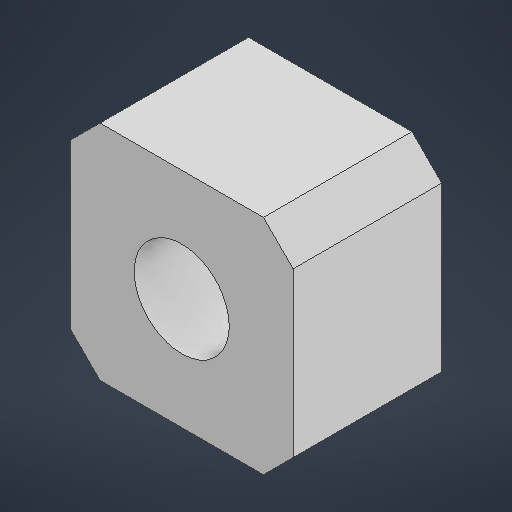
# Autodesk Inventor part: EndEffector_holder_Touch
Saved by Autodesk Inventor 2025.2 (Build 292293000, 293)
## iProperties
Created: 2025-07-03
Part Number: EndEffector_holder_Touch
Material: Generic
Document SubType Name: Modeling
Designer: Tiago
Density: 1 g/cm^3
Appearance: Default
Author: Tiago
Autodesk Inventor part; units mm, degrees
ref_plane "YZ Plane" through (0, 0, 0) normal (1, 0, 0) x (0, 1, 0)
ref_plane "XZ Plane" through (0, 0, 0) normal (0, 1, 0) x (-1, 0, 0)
ref_plane "XY Plane" through (0, 0, 0) normal (0, 0, 1) x (1, 0, 0)
sketch "Sketch1" plane through (0, 0, 0) normal (0, 0, 1) x (1, 0, 0)
  circle A0 centre (0, 0) radius 1.6
  line L0 (-3.75, -3.75) -> (3.75, -3.75)
  line L1 (3.75, -3.75) -> (3.75, 3.75)
  line L2 (3.75, 3.75) -> (-3.75, 3.75)
  line L3 (-3.75, 3.75) -> (-3.75, -3.75)
  point P0 (3.75, 0)
  point P1 (0, 3.75)
  dimension "d0" = 3.2
  dimension "d1" = 7.5
  dimension "d2" = 7.5
  constraints: 8 end point, 2 midpoint, 2 parallel, 1 centre point, 1 coincident, 1 horizontal, 1 horizontal alignment, 1 perpendicular, 1 vertical alignment
  measures "d0" diameter of A0
  measures "d1" distance of L0.end L1.end
  measures "d2" distance of L1.end L2.end
extrude "Extrusion1" add sketch "Sketch1" along normal blind 5
chamfer "Chamfer1" distance 1 angle 45 4 edges at (3.75, -3.75, 2.5) (-3.75, -3.75, 2.5) (-3.75, 3.75, 2.5) (3.75, 3.75, 2.5)
body "Solid1"
